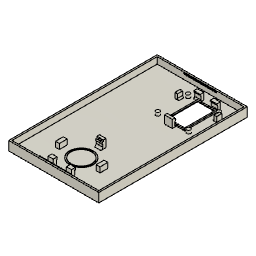
Outer Case Top v33 (Autodesk Fusion 360 design; units mm, degrees)
Autodesk Fusion 360 part; units mm, degrees
sketch "Sketch2" plane through (0, 0, 0) normal (0, 0, 1) x (1, 0, 0)
  line L0 (0, 0) -> (69.4, 0)
  line L1 (69.4, 0) -> (69.4, 114.4)
  line L2 (69.4, 114.4) -> (0, 114.4)
  line L3 (0, 114.4) -> (0, 0)
  dimension "d135" = 114.4
  dimension "d136" = 69.4
  constraint horizontal L0
  constraint vertical L1
  constraint horizontal L2
  constraint vertical L3
  constraint coincident L0.start L3.end
  measures "d135" distance of L0.start L2.end
  measures "d136" distance of L0.start L0.end
extrude "Extrude4" add sketch "Sketch2" along normal blind 2
sketch "Sketch3" plane through (0, 0, 2) normal (0, 0, 1) x (-1, 0, 0)
  line L0 (0, -114.4) -> (0, 0)
  line L1 (0, 0) -> (-69.4, 0)
  line L2 (-69.4, 0) -> (-69.4, -114.4)
  line L3 (-69.4, -114.4) -> (0, -114.4)
  circle A0 centre (-35.15, -103.09) radius 1.5
  circle A1 centre (-35.15, -79.71) radius 1.5
  circle A2 centre (-58.95, -103.09) radius 1.5
  circle A3 centre (-58.95, -79.71) radius 1.5
  line L4 (-38.15, -105.09) -> (-43.15, -105.09)
  line L5 (-43.15, -105.09) -> (-43.15, -107.09)
  line L6 (-43.15, -107.09) -> (-38.15, -107.09)
  line L7 (-38.15, -107.09) -> (-38.15, -105.09)
  line L8 (-50.95, -105.09) -> (-55.95, -105.09)
  line L9 (-55.95, -105.09) -> (-55.95, -107.09)
  line L10 (-55.95, -107.09) -> (-50.95, -107.09)
  line L11 (-50.95, -107.09) -> (-50.95, -105.09)
  line L12 (-44.05, -75.96) -> (-50.05, -75.96)
  line L13 (-50.05, -75.96) -> (-50.05, -77.96)
  line L14 (-50.05, -77.96) -> (-44.05, -77.96)
  line L15 (-44.05, -77.96) -> (-44.05, -75.96)
  line L16 (-42.45, -103.15) -> (-55.45, -103.15)
  line L17 (-55.45, -103.15) -> (-55.45, -80.15)
  line L18 (-55.45, -80.15) -> (-42.45, -80.15)
  line L19 (-42.45, -80.15) -> (-42.45, -103.15)
  line L20 (-56.45, -104.15) -> (-56.45, -79.15)
  line L21 (-56.45, -79.15) -> (-41.45, -79.15)
  line L22 (-41.45, -79.15) -> (-41.45, -104.15)
  line L23 (-41.45, -104.15) -> (-56.45, -104.15)
  line L24 (-1.25, -1.25) -> (-68.15, -1.25)
  line L25 (-68.15, -1.25) -> (-68.15, -113.15)
  line L26 (-68.15, -113.15) -> (-1.25, -113.15)
  line L27 (-1.25, -113.15) -> (-1.25, -1.25)
  line L28 (-25.675, -4.675) -> (-29.675, -4.675)
  line L29 (-29.675, -4.675) -> (-29.675, -7.175)
  line L30 (-29.675, -7.175) -> (-25.675, -7.175)
  line L31 (-25.675, -7.175) -> (-25.675, -4.675)
  line L32 (-39.725, -4.675) -> (-43.725, -4.675)
  line L33 (-43.725, -4.675) -> (-43.725, -7.175)
  line L34 (-43.725, -7.175) -> (-39.725, -7.175)
  line L35 (-39.725, -7.175) -> (-39.725, -4.675)
  line L36 (-32.2, -35.275) -> (-37.2, -35.275)
  line L37 (-37.2, -35.275) -> (-37.2, -37.775)
  line L38 (-37.2, -37.775) -> (-32.2, -37.775)
  line L39 (-32.2, -37.775) -> (-32.2, -35.275)
  line L40 (-48.85, -24.5) -> (-51.85, -24.5)
  line L41 (-51.85, -24.5) -> (-51.85, -18.5)
  line L42 (-51.85, -18.5) -> (-48.85, -18.5)
  line L43 (-48.85, -18.5) -> (-48.85, -24.5)
  line L44 (-17.55, -24.5) -> (-20.55, -24.5)
  line L45 (-20.55, -24.5) -> (-20.55, -18.5)
  line L46 (-20.55, -18.5) -> (-17.55, -18.5)
  line L47 (-17.55, -18.5) -> (-17.55, -24.5)
  circle A4 centre (-34.7, -21.25) radius 8.0623
  circle A5 centre (-34.7, -21.25) radius 9.0623
  line L48 (0, 0) -> (-69.4, 0)
  line L49 (0, -114.4) -> (0, 0)
  line L50 (-31, -110) -> (-68.15, -110)
  line L51 (-68.15, -110) -> (-68.15, -72)
  line L52 (-31, -72) -> (-31, -110)
  line L53 (-13, -40.0481) -> (-56, -40.0481)
  line L54 (-56, -40.0481) -> (-56, -2.3932)
  line L55 (-56, -2.3932) -> (-13, -2.3932)
  line L56 (-13, -2.3932) -> (-13, -40.0481)
  line L57 (-63.15, -101.09) -> (-61.15, -101.09)
  line L58 (-61.15, -101.09) -> (-61.15, -97.09)
  line L59 (-61.15, -97.09) -> (-63.15, -97.09)
  line L60 (-63.15, -97.09) -> (-63.15, -101.09)
  line L61 (-30.95, -101.09) -> (-32.95, -101.09)
  line L62 (-32.95, -101.09) -> (-32.95, -97.09)
  line L63 (-32.95, -97.09) -> (-30.95, -97.09)
  line L64 (-30.95, -97.09) -> (-30.95, -101.09)
  line L65 (-68.15, -72) -> (-31, -72)
  dimension "d33" = 3
  dimension "d34" = 3
  dimension "d35" = 3
  dimension "d36" = 3
  dimension "d37" = 23.38
  dimension "d38" = 23.8
  dimension "d39" = 5
  dimension "d40" = 2
  dimension "d41" = 5
  dimension "d42" = 2
  dimension "d45" = 6
  dimension "d46" = 2
  dimension "d47" = 2
  dimension "d50" = 3
  dimension "d51" = 3
  dimension "d52" = 23
  dimension "d53" = 13
  dimension "d54" = 2.19
  dimension "d55" = 3.5
  dimension "d56" = -1
  dimension "d82" = -1.25
  dimension "d86" = 10
  dimension "d87" = 4
  dimension "d88" = 2.5
  dimension "d89" = 4
  dimension "d90" = 2.5
  dimension "d93" = 5
  dimension "d94" = 2.5
  dimension "d96" = 3
  dimension "d97" = 6
  dimension "d98" = 3
  dimension "d99" = 6
  dimension "d102" = 11.65
  dimension "d103" = 28.3
  dimension "d104" = 1
  dimension "d122" = 14.15
  dimension "d129" = 57
  dimension "d131" = 20
  dimension "d137" = 69.4
  dimension "d138" = 34.7
  dimension "d149" = 2
  dimension "d150" = 4
  dimension "d151" = 2.2
  dimension "d152" = 2
  dimension "d153" = 2
  dimension "d154" = 4
  dimension "d155" = 2
  dimension "d156" = 2.2
  dimension "d165" = 8.9
  dimension "d169" = 28.1
  dimension "d170" = 14.025
  dimension "d193" = 114.4
  dimension "d205" = 5
  constraint vertical A0.centre A1.centre
  constraint horizontal A0.centre A2.centre
  constraint vertical A2.centre A3.centre
  constraint horizontal A1.centre A3.centre
  constraint horizontal L4
  constraint vertical L5
  constraint horizontal L6
  constraint vertical L7
  constraint horizontal L8
  constraint vertical L9
  constraint horizontal L10
  constraint vertical L11
  constraint horizontal L12
  constraint vertical L13
  constraint horizontal L14
  constraint vertical L15
  constraint horizontal L4.start L8.start
  constraint horizontal L16
  constraint vertical L17
  constraint horizontal L18
  constraint vertical L19
  constraint horizontal L28
  constraint vertical L29
  constraint horizontal L30
  constraint vertical L31
  constraint horizontal L32
  constraint vertical L33
  constraint horizontal L34
  constraint vertical L35
  constraint horizontal L36
  constraint vertical L37
  constraint horizontal L38
  constraint vertical L39
  constraint horizontal L30.end L34.end
  constraint horizontal L40
  constraint vertical L41
  constraint horizontal L42
  constraint vertical L43
  constraint horizontal L44
  constraint vertical L45
  constraint horizontal L46
  constraint vertical L47
  constraint horizontal L40.start L44.end
  constraint horizontal L50
  constraint vertical L51
  constraint vertical L52
  constraint horizontal L53
  constraint vertical L54
  constraint horizontal L55
  constraint vertical L56
  constraint horizontal L57
  constraint vertical L58
  constraint horizontal L59
  constraint vertical L60
  constraint horizontal L61
  constraint vertical L62
  constraint horizontal L63
  constraint vertical L64
  constraint coincident L25 L51.end
  constraint perpendicular L52 L65
  measures "d33" diameter of A0
  measures "d34" diameter of A1
  measures "d35" diameter of A2
  measures "d36" diameter of A3
  measures "d37" distance of A0.centre A1.centre
  measures "d38" distance of A0.centre A2.centre
  measures "d39" distance of L4.start L4.end
  measures "d40" distance of L4.start L6.end
  measures "d41" distance of L8.start L8.end
  measures "d42" distance of L8.start L10.end
  measures "d45" distance of L12.start L12.end
  measures "d46" distance of L12.start L14.end
  measures "d47" distance of A0.centre L4
  measures "d50" distance of A0.centre L7
  measures "d51" distance of A2.centre L9
  measures "d52" distance of L16.start L18.end
  measures "d53" distance of L17 L19
  measures "d54" distance of L14 L18
  measures "d55" distance of A3.centre L17
  measures "d86" distance of L16 L26
  measures "d87" distance of L28.start L28.end
  measures "d88" distance of L28.start L30.end
  measures "d89" distance of L32.start L32.end
  measures "d90" distance of L32.start L34.end
  measures "d93" distance of L36.start L36.end
  measures "d94" distance of L36.start L38.end
  measures "d96" distance of L40.start L40.end
  measures "d97" distance of L40.start L42.end
  measures "d98" distance of L44.start L44.end
  measures "d99" distance of L44.start L46.end
  measures "d102" distance of L37 L43
  measures "d103" distance of L43 L45
  measures "d122" distance of L45 A4.centre
  measures "d131" distance of L24 A4.centre
  measures "d137" distance of L0.end L1.end
  measures "d138" distance of A4.centre L49
  measures "d149" distance of L57.start L57.end
  measures "d150" distance of L57.start L59.end
  measures "d151" distance of A2.centre L58
  measures "d152" distance of A2.centre L57
  measures "d153" distance of L61.start L61.end
  measures "d154" distance of L61.start L63.end
  measures "d155" distance of A0.centre L61
  measures "d156" distance of A0.centre L62
  measures "d165" distance of A1.centre L15
  measures "d169" distance of L34 L36
  measures "d170" distance of L36 A4.centre
  measures "d193" distance of L0.start L0.end
  measures "d205" distance of L25 L60
extrude "Extrude17" add sketch "Sketch3" along normal blind 4 contours L52 L61 L63 L64 | L52 L61 L62 L63 | L57 L58 L59 L60
extrude "Extrude15" cut sketch "Sketch3" against normal blind 3 contours L16 L17 L18 L19
extrude "Extrude11" add sketch "Sketch3" along normal blind 0.3 contours A5
extrude "Extrude12" add sketch "Sketch3" along normal blind 4 contours L40 L41 L42 L43 | L44 L45 L46 L47
extrude "Extrude13" add sketch "Sketch3" along normal blind 3.23 contours L28 L29 L30 L31 | L32 L33 L34 L35 | L36 L37 L38 L39
sketch "Sketch7" plane through (0, 0, 5.23) normal (0, 0, 1) x (-1, 0, 0)
  line L0 (-32.2, -37.775) -> (-37.2, -37.775)
  line L1 (-37.2, -37.775) -> (-37.2, -34.775)
  line L2 (-37.2, -34.775) -> (-32.2, -34.775)
  line L3 (-32.2, -34.775) -> (-32.2, -37.775)
  line L4 (-25.675, -4.675) -> (-29.675, -4.675)
  line L5 (-29.675, -4.675) -> (-29.675, -7.675)
  line L6 (-29.675, -7.675) -> (-25.675, -7.675)
  line L7 (-25.675, -7.675) -> (-25.675, -4.675)
  line L8 (-39.725, -4.675) -> (-43.725, -4.675)
  line L9 (-43.725, -4.675) -> (-43.725, -7.675)
  line L10 (-43.725, -7.675) -> (-39.725, -7.675)
  line L11 (-39.725, -7.675) -> (-39.725, -4.675)
  line L12 (-32.2, -37.775) -> (-32.2, -35.275)
  line L13 (-32.2, -35.275) -> (-37.2, -35.275)
  line L14 (-37.2, -35.275) -> (-37.2, -37.775)
  line L15 (-37.2, -37.775) -> (-32.2, -37.775)
  line L16 (-39.725, -7.175) -> (-39.725, -4.675)
  line L17 (-39.725, -4.675) -> (-43.725, -4.675)
  line L18 (-43.725, -4.675) -> (-43.725, -7.175)
  line L19 (-43.725, -7.175) -> (-39.725, -7.175)
  line L20 (-25.675, -7.175) -> (-25.675, -4.675)
  line L21 (-25.675, -4.675) -> (-29.675, -4.675)
  line L22 (-29.675, -4.675) -> (-29.675, -7.175)
  line L23 (-29.675, -7.175) -> (-25.675, -7.175)
  point P0 (-32.2, -37.775)
  point P1 (-25.675, -4.675)
  point P2 (-39.725, -4.675)
  point P3 (-37.2, -37.775)
  dimension "d112" = 3
  dimension "d113" = 4
  dimension "d114" = 3
  dimension "d115" = 4
  dimension "d116" = 3
  constraint horizontal L0
  constraint vertical L1
  constraint horizontal L2
  constraint vertical L3
  constraint horizontal L4
  constraint vertical L5
  constraint horizontal L6
  constraint vertical L7
  constraint horizontal L8
  constraint vertical L9
  constraint horizontal L10
  constraint vertical L11
  constraint coincident P0 L0.start
  constraint coincident P1 L4.start
  constraint coincident P2 L8.start
  constraint coincident P3 L0.end
  measures "d112" distance of P0 L2.end
  measures "d113" distance of P1 L4.end
  measures "d114" distance of P1 L6.end
  measures "d115" distance of P2 L8.end
  measures "d116" distance of P2 L10.end
extrude "Extrude14" add sketch "Sketch7" along normal blind 1.8
extrude "Extrude10" add sketch "Sketch3" along normal blind 5 contours L0 L1 L2 L3 L48 L49
extrude "Extrude9" add sketch "Sketch3" along normal blind 1 contours L20 L21 L22 L23
extrude "Extrude6" add sketch "Sketch3" along normal blind 3.63 contours L4 L5 L6 L7 | L8 L9 L10 L11 | L12 L13 L14 L15
extrude "Extrude5" add sketch "Sketch3" along normal blind 2.34 contours A0 | A1 | A2 | A3
sketch "Sketch6" plane through (0, 0, 5.63) normal (0, 0, 1) x (-1, 0, 0)
  line L0 (-38.15, -107.09) -> (-38.15, -105.09)
  line L1 (-38.15, -105.09) -> (-43.15, -105.09)
  line L2 (-43.15, -105.09) -> (-43.15, -107.09)
  line L3 (-43.15, -107.09) -> (-38.15, -107.09)
  line L4 (-38.15, -107.09) -> (-43.15, -107.09)
  line L5 (-43.15, -107.09) -> (-43.15, -104.39)
  line L6 (-43.15, -104.39) -> (-38.15, -104.39)
  line L7 (-38.15, -104.39) -> (-38.15, -107.09)
  line L8 (-50.95, -107.09) -> (-55.95, -107.09)
  line L9 (-55.95, -107.09) -> (-55.95, -104.39)
  line L10 (-55.95, -104.39) -> (-50.95, -104.39)
  line L11 (-50.95, -104.39) -> (-50.95, -107.09)
  line L12 (-44.05, -75.96) -> (-50.05, -75.96)
  line L13 (-50.05, -75.96) -> (-50.05, -78.66)
  line L14 (-50.05, -78.66) -> (-44.05, -78.66)
  line L15 (-44.05, -78.66) -> (-44.05, -75.96)
  point P0 (-50.95, -107.09)
  point P1 (-44.05, -75.96)
  point P2 (-50.05, -75.96)
  dimension "d68" = 2.7
  dimension "d69" = 5
  dimension "d70" = 2.7
  dimension "d74" = 2.7
  dimension "d123" = 5
  constraint horizontal L4
  constraint vertical L5
  constraint horizontal L6
  constraint vertical L7
  constraint coincident L0.start L3.end
  constraint horizontal L8
  constraint vertical L9
  constraint horizontal L10
  constraint vertical L11
  constraint horizontal L12
  constraint vertical L13
  constraint horizontal L14
  constraint vertical L15
  constraint coincident P0 L8.start
  constraint coincident P1 L12.start
  constraint vertical P2 L12.end
  measures "d68" distance of L0.start L6.end
  measures "d69" distance of P0 L8.end
  measures "d70" distance of P0 L10.end
  measures "d74" distance of P1 L14.end
  measures "d123" distance of L5.end L6.end
extrude "Extrude8" add sketch "Sketch6" along normal blind 1.5
chamfer "Chamfer1" distance 0.7 angle 45 3 edges at (40.65, 104.39, 5.63) (53.45, 104.39, 5.63) (47.05, 78.66, 5.63)
fillet "Fillet1" radius 1 3 edges at (47.05, 77.96, 2) (53.45, 105.09, 2) (40.65, 105.09, 2)
fillet "Fillet1" radius 1 2 edges at (61.15, 99.09, 2) (32.95, 99.09, 2)
chamfer "Chamfer4" distance 2.5 angle 45 4 edges at (48.95, 103.15, 0) (55.45, 91.65, 0) (42.45, 91.65, 0) (48.95, 80.15, 0)
chamfer "Chamfer5" distance 0.5 angle 45 3 edges at (34.7, 34.775, 5.23) (27.675, 7.675, 5.23) (41.725, 7.675, 5.23)
sketch "Sketch8" plane through (0, 0, 0) normal (0, 0, -1) x (1, 0, 0)
  line L0 (0, 0) -> (0, -114.4)
  line L1 (0, -114.4) -> (69.4, -114.4)
  line L2 (69.4, -114.4) -> (69.4, 0)
  line L3 (69.4, 0) -> (0, 0)
  line L4 (57.95, -77.65) -> (57.95, -105.65)
  line L5 (57.95, -105.65) -> (39.95, -105.65)
  line L6 (39.95, -105.65) -> (39.95, -77.65)
  line L7 (39.95, -77.65) -> (57.95, -77.65)
  line L8 (12.8279, -10.7958) -> (12.8279, -104.0301) construction
  line L9 (12.8279, -104.0301) -> (24.8279, -104.0301) construction
  line L10 (24.8279, -104.0301) -> (24.8279, -10.7958) construction
  line L11 (24.8279, -10.7958) -> (12.8279, -10.7958) construction
  text T0 "Ferg Data Logger" font "Arial" height 12 align ink ink in box 0 x 0 at (12.8279, -10.7958) x (0, -1) y (1, 0) spacing 1 height is em
  constraint perpendicular L8 L9
  constraint parallel L8 L10
  constraint parallel L9 L11
extrude "Extrude16" cut sketch "Sketch8" against normal blind 0.5 text T0
sketch "Sketch10" plane through (0, 113.15, 0) normal (0, -1, 0) x (1, 0, 0)
  line L0 (1.25, 2) -> (68.15, 2)
  line L1 (68.15, 2) -> (68.15, 7)
  line L2 (68.15, 7) -> (1.25, 7)
  line L3 (1.25, 7) -> (1.25, 2)
  line L4 (21.95, 7) -> (46.95, 7)
  line L5 (46.95, 7) -> (46.95, 5.6)
  line L6 (46.95, 5.6) -> (21.95, 5.6)
  line L7 (21.95, 5.6) -> (21.95, 7)
  dimension "d139" = 25
  dimension "d140" = 1.4
  dimension "d141" = 66.4
  dimension "d142" = 20.7
  constraint horizontal L4
  constraint vertical L5
  constraint horizontal L6
  constraint vertical L7
  constraint coincident L2 L4.start
  measures "d139" distance of L4.start L4.end
  measures "d140" distance of L4.start L6.end
  measures "d142" distance of L3 L7
revolve "Revolve1" add sketch "Sketch10" angle 25 about axis through (46.95, 113.15, 5.6) along (1, 0, 0) contours L2 L4 L5 L6 L7
sketch "Sketch11" plane through (0, 1.25, 0) normal (0, 1, 0) x (-1, 0, 0)
  line L0 (-68.15, 2) -> (-1.25, 2)
  line L1 (-1.25, 2) -> (-1.25, 7)
  line L2 (-1.25, 7) -> (-68.15, 7)
  line L3 (-46.95, 7) -> (-21.95, 7)
  line L4 (-21.95, 7) -> (-21.95, 5.6)
  line L5 (-21.95, 5.6) -> (-46.95, 5.6)
  line L6 (-46.95, 5.6) -> (-46.95, 7)
  line L7 (-68.15, 7) -> (-68.15, 2)
  dimension "d144" = 25
  dimension "d145" = 1.4
  dimension "d146" = 66.4
  dimension "d147" = 20.7
  constraint horizontal L3
  constraint vertical L4
  constraint horizontal L5
  constraint vertical L6
  constraint coincident L2 L3.start
  measures "d144" distance of L3.start L3.end
  measures "d145" distance of L3.start L5.end
  measures "d147" distance of L1 L4
revolve "Revolve2" add sketch "Sketch11" angle 25 about axis through (21.95, 1.25, 5.6) along (-1, 0, 0) contours L2 L3 L4 L5 L6
sketch "Sketch12" plane through (0, 0, 7.03) normal (0, 0, 1) x (-1, 0, 0)
  line L0 (-32.2, -34.775) -> (-37.2, -34.775)
  line L1 (-37.2, -34.775) -> (-37.2, -37.775)
  line L2 (-37.2, -37.775) -> (-32.2, -37.775)
  line L3 (-32.2, -37.775) -> (-32.2, -34.775)
  line L4 (-32.2, -37.775) -> (-37.2, -37.775)
  line L5 (-37.2, -37.775) -> (-37.2, -35.775)
  line L6 (-37.2, -35.775) -> (-32.2, -35.775)
  line L7 (-32.2, -35.775) -> (-32.2, -37.775)
  dimension "d160" = 2
  constraint horizontal L4
  constraint vertical L5
  constraint horizontal L6
  constraint vertical L7
  constraint coincident L2.end L3.start
  constraint coincident L1.end L2.start
  measures "d160" distance of L2.end L6.end
extrude "Extrude18" add sketch "Sketch12" along normal blind 1 contours L1 L2 L3 L4 L5 L6 L7
sketch "Sketch13" plane through (0, 0, 7.13) normal (0, 0, 1) x (-1, 0, 0)
  line L0 (-44.05, -78.66) -> (-44.05, -75.96)
  line L1 (-44.05, -75.96) -> (-50.05, -75.96)
  line L2 (-50.05, -75.96) -> (-50.05, -78.66)
  line L3 (-50.05, -78.66) -> (-44.05, -78.66)
  line L4 (-50.05, -77.96) -> (-44.05, -77.96)
  line L5 (-44.05, -77.96) -> (-44.05, -75.96)
  line L6 (-44.05, -75.96) -> (-50.05, -75.96)
  line L7 (-50.05, -75.96) -> (-50.05, -77.96)
  dimension "d166" = 2
  constraint horizontal L4
  constraint vertical L5
  constraint horizontal L6
  constraint vertical L7
  constraint coincident L0.end L1.start
  constraint coincident L2 L4.start
  measures "d166" distance of L4.start L1.end
extrude "Extrude19" add sketch "Sketch13" along normal blind 1 contours L0 L1 L2 L4 L5 L6 L7
fillet "Fillet3" radius 1.5 1 edges at (34.7, 35.275, 2)
sketch "Sketch18" plane through (0, 0, 2) normal (0, 0, 1) x (-1, 0, 0)
  line L0 (-32.2, -33.775) -> (-32.2, -37.775)
  line L1 (-32.2, -37.775) -> (-37.2, -37.775)
  line L2 (-37.2, -37.775) -> (-37.2, -33.775)
  line L3 (-37.2, -33.775) -> (-32.2, -33.775)
  line L4 (-33.95, -97.09) -> (-30.95, -97.09)
  line L5 (-30.95, -97.09) -> (-30.95, -101.09)
  line L6 (-30.95, -101.09) -> (-33.95, -101.09)
  line L7 (-33.95, -101.09) -> (-33.95, -97.09)
  line L8 (-60.15, -101.09) -> (-63.15, -101.09)
  line L9 (-63.15, -101.09) -> (-63.15, -97.09)
  line L10 (-63.15, -97.09) -> (-60.15, -97.09)
  line L11 (-60.15, -97.09) -> (-60.15, -101.09)
  line L12 (-50.05, -78.96) -> (-50.05, -75.96)
  line L13 (-50.05, -75.96) -> (-44.05, -75.96)
  line L14 (-44.05, -75.96) -> (-44.05, -78.96)
  line L15 (-44.05, -78.96) -> (-50.05, -78.96)
  circle A0 centre (-58.95, -103.09) radius 1.5
  circle A1 centre (-35.15, -103.09) radius 1.5
  circle A2 centre (-58.95, -79.71) radius 1.5
  circle A3 centre (-35.15, -79.71) radius 1.5
  line L16 (-41.45, -104.09) -> (-38.15, -104.09)
  line L17 (-38.15, -104.09) -> (-38.15, -107.09)
  line L18 (-38.15, -107.09) -> (-43.15, -107.09)
  line L19 (-43.15, -107.09) -> (-43.15, -104.15)
  line L20 (-43.15, -104.15) -> (-50.95, -104.15)
  line L21 (-50.95, -104.15) -> (-50.95, -107.09)
  line L22 (-50.95, -107.09) -> (-55.95, -107.09)
  line L23 (-55.95, -107.09) -> (-55.95, -104.15)
  line L24 (-55.95, -104.15) -> (-56.45, -104.15)
  line L25 (-56.45, -104.15) -> (-56.45, -79.15)
  line L26 (-56.45, -79.15) -> (-41.45, -79.15)
  line L27 (-41.45, -79.15) -> (-41.45, -104.09)
  line L28 (-1.25, -1.25) -> (-68.15, -1.25)
  line L29 (-68.15, -1.25) -> (-68.15, -113.15)
  line L30 (-68.15, -113.15) -> (-1.25, -113.15)
  line L31 (-1.25, -113.15) -> (-1.25, -1.25)
  line L32 (-39.725, -7.175) -> (-43.725, -7.175)
  line L33 (-43.725, -7.175) -> (-43.725, -4.675)
  line L34 (-43.725, -4.675) -> (-39.725, -4.675)
  line L35 (-39.725, -4.675) -> (-39.725, -7.175)
  line L36 (-25.675, -7.175) -> (-29.675, -7.175)
  line L37 (-29.675, -7.175) -> (-29.675, -4.675)
  line L38 (-29.675, -4.675) -> (-25.675, -4.675)
  line L39 (-25.675, -4.675) -> (-25.675, -7.175)
  line L40 (-48.85, -18.5) -> (-48.85, -24.5)
  line L41 (-48.85, -24.5) -> (-51.85, -24.5)
  line L42 (-51.85, -24.5) -> (-51.85, -18.5)
  line L43 (-51.85, -18.5) -> (-48.85, -18.5)
  line L44 (-17.55, -18.5) -> (-17.55, -24.5)
  line L45 (-17.55, -24.5) -> (-20.55, -24.5)
  line L46 (-20.55, -24.5) -> (-20.55, -18.5)
  line L47 (-20.55, -18.5) -> (-17.55, -18.5)
  circle A4 centre (-34.7, -21.25) radius 9.0623
  line L48 (-5.2392, -108.6182) -> (-65.3716, -108.6182)
  line L49 (-65.3716, -108.6182) -> (-65.3716, -3.4636)
  line L50 (-65.3716, -3.4636) -> (-5.2392, -3.4636)
  line L51 (-5.2392, -3.4636) -> (-5.2392, -108.6182)
  constraint horizontal L48
  constraint vertical L49
  constraint horizontal L50
  constraint vertical L51
extrude "Extrude22" [suppressed]
equation "d34 = d33"
equation "d35 = d33"
equation "d36 = d33"
equation "d42 = d40"
equation "d46 = d40"
equation "d51 = d50"
equation "d68 = d70"
equation "d74 = d70"
equation "d87 = d89"
equation "d88 = d94"
equation "d90 = d94"
equation "d96 = d98"
equation "d97 = d99"
equation "d102 = ( d103 - d93 ) / 2"
equation "d109 = 2.93 mm + 0.3 mm"
equation "d112 = d114"
equation "d115 = d113"
equation "d116 = d114"
equation "d122 = d103 / 2"
equation "d123 = d69"
equation "d138 = 69.40 mm / 2"
equation "d142 = ( 66.40 mm - d139 ) / 2"
equation "d147 = ( 66.40 mm - d144 ) / 2"
equation "d165 = ( d38 - d45 ) / 2"
